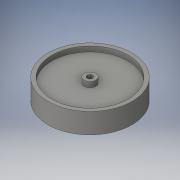
# Autodesk Inventor part: Wheel Hub
Saved by Autodesk Inventor 2016 (Build 200138000, 138)
## iProperties
Created: 2018-04-26
Part Number: Wheel Hub
Material: Acetal Resin, Black
Document SubType Name: Modeling
Designer: 2000083068
Density: 1.425 g/cm^3
Appearance: Smooth - Medium Gray
Mass: 36.1545 g
Surface Area: 97.592 cm^2
Volume: 36.1545 cm^3
Author: 2000083068
Autodesk Inventor part; units mm, degrees
ref_plane "YZ Plane" through (0, 0, 0) normal (1, 0, 0) x (0, 1, 0)
ref_plane "XZ Plane" through (0, 0, 0) normal (0, 1, 0) x (-1, 0, 0)
ref_plane "XY Plane" through (0, 0, 0) normal (0, 0, 1) x (1, 0, 0)
sketch "Sketch1" plane through (0, 0, 0) normal (0, 1, 0) x (-1, 0, 0)
  line L0 (18.3309, -0.0019) -> (9.1638, -15.8759)
  line L1 (9.1638, -15.8759) -> (-9.1671, -15.8741)
  line L2 (-9.1671, -15.8741) -> (-18.3309, 0.0019)
  line L3 (-18.3309, 0.0019) -> (-9.1638, 15.8759)
  line L4 (-9.1638, 15.8759) -> (9.1671, 15.8741)
  line L5 (9.1671, 15.8741) -> (18.3309, -0.0019)
  point P0 (0, 0)
  dimension "d2" = 31.75
  constraints: 12 end point, 13 other
  measures "d2" distance between parallel lines of L1 L4
extrude "Extrusion1" add sketch "Sketch1" along normal blind 30.1625
sketch "Sketch2" plane through (0, 30.1625, 0) normal (0, 1, 0) x (1, 0, 0)
  circle A0 centre (0, 0) radius 14.605
  dimension "d5" = 29.21
  constraints: 1 centre point, 1 coincident
  measures "d5" diameter of A0
extrude "Extrusion2" add sketch "Sketch2" along normal blind 13.4938
sketch "Sketch3" plane through (0, 0, 0) normal (0, -1, 0) x (1, 0, 0)
  circle A0 centre (0, 0) radius 14.605
  dimension "d8" = 29.21
  constraints: 1 centre point, 1 coincident
  measures "d8" diameter of A0
extrude "Extrusion3" add sketch "Sketch3" along normal blind 13.4938
sketch "Sketch4" plane through (0, 43.6562, 0) normal (0, 1, 0) x (1, 0, 0)
  line L0 (-7.479, 0) -> (-3.7395, 6.477)
  line L1 (-3.7395, 6.477) -> (3.7395, 6.477)
  line L2 (3.7395, 6.477) -> (7.479, 0)
  line L3 (7.479, 0) -> (3.7395, -6.477)
  line L4 (3.7395, -6.477) -> (-3.7395, -6.477)
  line L5 (-3.7395, -6.477) -> (-7.479, 0)
  point P0 (0, 0)
  point P1 (0, 0)
  dimension "d11" = 12.954
  constraints: 12 end point, 1 coincident, 13 other
  measures "d11" distance between parallel lines of L1 L4
extrude "Extrusion4" cut sketch "Sketch4" against normal through all
fillet "Fillet1" radius 1.524 6 edges at (7.479, 15.0813, 0) (3.7395, 15.0813, -6.477) (-7.479, 15.0813, 0) (-3.7395, 15.0813, -6.477) (-3.7395, 15.0813, 6.477) (3.7395, 15.0813, 6.477)
sketch "Sketch5" plane through (0, 30.1625, 0) normal (0, 1, 0) x (1, 0, 0)
  circle A0 centre (0, 0) radius 14.8083
  circle A1 centre (0, 0) radius 95.25
  dimension "d15" = 190.5
  constraints: 2 centre point, 2 coincident
  measures "d15" diameter of A1
extrude "Extrusion5" add sketch "Sketch5" against normal blind 30.226
sketch "Sketch6" plane through (0, 30.1625, 0) normal (0, 1, 0) x (1, 0, 0)
  circle A0 centre (0, 0) radius 95.25
  circle A1 centre (0, 0) radius 104.775
  dimension "d18" = 209.55
  constraints: 2 centre point, 2 coincident
  measures "d18" diameter of A1
extrude "Extrusion6" add sketch "Sketch6" along normal blind 12.7 and the other way blind 38.1
body "Solid1"
